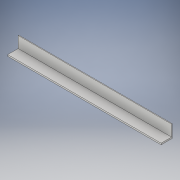
# Autodesk Inventor part: Shutter
Saved by Autodesk Inventor 2019.3 (Build 233278000, 278)
## iProperties
Created: 2020-10-08
Part Number: Shutter
Material: Generisch
Document SubType Name: Modeling
Designer: Nicolas Frick
Density: 1 g/cm^3
Appearance: Vorgabe
Author: Nicolas Frick
Autodesk Inventor part; units mm, degrees
ref_plane "YZ Plane" through (0, 0, 0) normal (1, 0, 0) x (0, 1, 0)
ref_plane "XZ Plane" through (0, 0, 0) normal (0, 1, 0) x (-1, 0, 0)
ref_plane "XY Plane" through (0, 0, 0) normal (0, 0, 1) x (1, 0, 0)
sketch "Skizze1" plane through (0, 0, 0) normal (0, 0, 1) x (1, 0, 0)
  line L0 (-102.4, 1) -> (102.4, 1)
  line L1 (102.4, 1) -> (102.4, -1)
  line L2 (102.4, -1) -> (-102.4, -1)
  line L3 (-102.4, -1) -> (-102.4, 1)
  line L4 (-102.4, 1) -> (102.4, -1) construction
  line L5 (102.4, 1) -> (-102.4, -1) construction
  point P0 (0, 0)
  dimension "d0" = 204.8
  dimension "d1" = 2
  constraints: 12 end point, 2 midpoint, 2 parallel, 1 horizontal, 1 perpendicular
  measures "d0" distance of L1.end L2.end
  measures "d1" distance of L0.end L1.end
extrude "Extrusion1" add sketch "Skizze1" along normal blind 15
sketch "Skizze2" plane through (-102.4, 1, 0) normal (0, 1, 0) x (1, 0, 0)
  line L0 (0, 0) -> (204.8, 0) projected
  line L1 (204.8, 0) -> (204.8, -15) projected
  line L2 (0, 0) -> (204.8, 0)
  line L3 (204.8, 0) -> (204.8, -1)
  line L4 (204.8, -1) -> (0, -1)
  line L5 (0, -1) -> (0, 0)
  point P0 (102.4, 0)
  dimension "d4" = 1
  constraints: 8 end point, 2 parallel, 1 horizontal, 1 perpendicular, 1 point on line
  measures "d4" distance of L2.end L3.end
extrude "Extrusion2" add sketch "Skizze2" along normal blind 15
